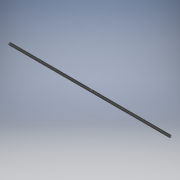
# Autodesk Inventor part: GBN1700MR2-90_info-1-13-13
Saved by Autodesk Inventor 2017.3 (Build 213256000, 256)
## iProperties
Part Number: GBN1700MR2-90_info-1-13-13
Material: Generic
Catalog Web Link: www.cadenas.de
Description: GBN__MR2-High Torque Timing Belts - MR2 Type
Vendor: MISUMI
Document SubType Name: Modeling
Designer: partserver
Manufacturer: MISUMI
Mass: 9.67395 g
Surface Area: 327.945 cm^2
Volume: 9.67395 cm^3
Density: 1 g/cm^3
Appearance: PSOLRGB-175-175-175
Category: PARTsolutions
Company: MISUMI
Title: GBN1700MR2-90
Author: Cadenas PARTsolutions
Comments: High Torque Timing Belts - MR2 Type
PSOL_IDENT_0: {$CADENAS_DATA\23d-libs\misumi\metric\48_timing_belts\gbn_mr2.prj},206 {VTYP=3D},{NB=GBN1700MR2-90_i
PSOL_IDENT_1: nfo-1-13-13},{LINA=GBN1700MR2-90},{NN=GBN__MR2},{DATE=08.06.2021 08:28:53},{GEOMDATE=10.03.2016 05:4
PSOL_IDENT_2: 5:00},{VERSION=},{LINEID=40},{WBVAR=NT,RSSP,NT1,NT2},{WBNUMERIC=NT,NT1,NT2}  {NB=GBN1700MR2-90_info-
PSOL_IDENT_3: 1-13-13},{LINA=GBN1700MR2-90},{KT=DUMMY},{PN=GBN1700MR2-90},{TYPE=GBN},{BNO=1700MR2},{BNW=9},{BNWALG=
PSOL_IDENT_4: 90},{NT=850},{BC=1700},{PITCH=2},{R1=0.15},{R2=1.00},{R3=0.555},{BB=0.40},{H=1.38},{HH=0.75},{II=0.6
PSOL_IDENT_5: 3},{PLD=0.254},{RSSP=1},{RSSPALG= '1','900 or Less','2','Over 900, 1200 or Less','3','Over 1200, 180
PSOL_IDENT_6: 0 or Less','4','Over 1800, 3600 or Less','5','Over 3600, 4800 or Less' },{NT1=13},{NT1ALG=13,14,15,1
PSOL_IDENT_7: 6,17,18,19,20,21,22,24,25,26,28,30,32,34,36,40,42,44,45,48,50,56,60,62,68,72},{NT2=13},{NT2ALG=13,14
PSOL_IDENT_8: ,15,16,17,18,19,20,21,22,24,25,26,28,30,32,34,36,40,42,44,45,48,50,56,60,62,68,72},{NT2ALG1=0},{NT2A
PSOL_IDENT_9: LG2=0},{NT2ALG3=13,14,15,16,17,18,19,20,21,22,24,25,26,28,30,32,34,36,40,42,44,45,48,50,56,60,62,68,
PSOL_IDENT_10: 72},{DRIVEP=8.27606},{DRP=7.77},{DRIVENP=8.27606},{DRNP=7.77},{BBCAL=3348.00000},{C=837.00},{NOTE=-}
PSOL_IDENT_11: ,{ASSCFGC=NT2,C},{ASSCFGCNOTE=-},{FS=0.00},{FL=0.00},{NT1SCR=16,18,20,22,23,24,25,26,28,30,32,34,36,
PSOL_IDENT_12: 40,44,48,50,60},{NT2SCR=0}
NB: GBN1700MR2-90_info-1-13-13
NN: GBN__MR2
NT: 850
NBSYN: $PN._info-$RSSP.-$NT1.-$NT2.
LINA: GBN1700MR2-90
CATALOG: Misumi
PN: GBN1700MR2-90
TYPE: GBN
BNO: 1700MR2
BNW: 9
BC: 1700
PITCH: 2
R1: 0.15
R2: 1
R3: 0.555
BB: 0.4
H: 1.38
HH: 0.75
II: 0.63
PLD: 0.254
RSSP: 900 or Less
NT1: 13
NT2: 13
SUPPLIER: MISUMI
ARTICLENO: GBN1700MR2-90_info-1-13-13
BOMINFO: GBN1700MR2-90
CREATOR: CADENAS GmbH
Autodesk Inventor part; units mm, degrees
ref_plane "YZ Plane" through (0, 0, 0) normal (1, 0, 0) x (0, 1, 0)
ref_plane "XZ Plane" through (0, 0, 0) normal (0, 1, 0) x (-1, 0, 0)
ref_plane "XY Plane" through (0, 0, 0) normal (0, 0, 1) x (1, 0, 0)
sketch "_____1" plane through (0, 0, 0) normal (0, 0, 1) x (1, 0, 0)
  arc A0 (0, 4.515) -> (0, -4.515) centre (0, 0) ccw
  line L0 (0, -4.515) -> (837, -4.515)
  arc A1 (837, -4.515) -> (837, 4.515) centre (837, 0) ccw
  line L1 (837, 4.515) -> (0, 4.515)
  arc A2 (0, 3.885) -> (0, -3.885) centre (0, 0) ccw
  line L2 (0, -3.885) -> (837, -3.885)
  arc A3 (837, -3.885) -> (837, 3.885) centre (837, 0) ccw
  line L3 (837, 3.885) -> (0, 3.885)
  constraints: 8 end point, 8 point on circle, 4 centre point
extrude "Extrusion1" add sketch "_____1" along normal mid plane 9
sketch "_____2" plane through (0, 0, 0) normal (0, 0, 1) x (1, 0, 0)
  line L0 (413.5, 4.515) -> (413.5, 3.885)
  line L1 (413.5, 3.885) -> (413.7598, 3.885)
  arc A0 (413.9085, 3.7546) -> (413.7598, 3.885) centre (413.7598, 3.735) ccw
  arc A1 (413.9085, 3.7546) -> (414.0011, 3.4468) centre (414.9, 3.885) ccw
  arc A2 (414.0011, 3.4468) -> (414.9989, 3.4468) centre (414.5, 3.69) ccw
  arc A3 (414.9989, 3.4468) -> (415.0915, 3.7546) centre (414.1, 3.885) ccw
  arc A4 (415.2402, 3.885) -> (415.0915, 3.7546) centre (415.2402, 3.735) ccw
  line L2 (415.2402, 3.885) -> (415.7598, 3.885)
  arc A5 (415.9085, 3.7546) -> (415.7598, 3.885) centre (415.7598, 3.735) ccw
  arc A6 (415.9085, 3.7546) -> (416.0011, 3.4468) centre (416.9, 3.885) ccw
  arc A7 (416.0011, 3.4468) -> (416.9989, 3.4468) centre (416.5, 3.69) ccw
  arc A8 (416.9989, 3.4468) -> (417.0915, 3.7546) centre (416.1, 3.885) ccw
  arc A9 (417.2402, 3.885) -> (417.0915, 3.7546) centre (417.2402, 3.735) ccw
  line L3 (417.2402, 3.885) -> (417.7598, 3.885)
  arc A10 (417.9085, 3.7546) -> (417.7598, 3.885) centre (417.7598, 3.735) ccw
  arc A11 (417.9085, 3.7546) -> (418.0011, 3.4468) centre (418.9, 3.885) ccw
  arc A12 (418.0011, 3.4468) -> (418.9989, 3.4468) centre (418.5, 3.69) ccw
  arc A13 (418.9989, 3.4468) -> (419.0915, 3.7546) centre (418.1, 3.885) ccw
  arc A14 (419.2402, 3.885) -> (419.0915, 3.7546) centre (419.2402, 3.735) ccw
  line L4 (419.2402, 3.885) -> (419.7598, 3.885)
  arc A15 (419.9085, 3.7546) -> (419.7598, 3.885) centre (419.7598, 3.735) ccw
  arc A16 (419.9085, 3.7546) -> (420.0011, 3.4468) centre (420.9, 3.885) ccw
  arc A17 (420.0011, 3.4468) -> (420.9989, 3.4468) centre (420.5, 3.69) ccw
  arc A18 (420.9989, 3.4468) -> (421.0915, 3.7546) centre (420.1, 3.885) ccw
  arc A19 (421.2402, 3.885) -> (421.0915, 3.7546) centre (421.2402, 3.735) ccw
  line L5 (421.2402, 3.885) -> (421.7598, 3.885)
  arc A20 (421.9085, 3.7546) -> (421.7598, 3.885) centre (421.7598, 3.735) ccw
  arc A21 (421.9085, 3.7546) -> (422.0011, 3.4468) centre (422.9, 3.885) ccw
  arc A22 (422.0011, 3.4468) -> (422.9989, 3.4468) centre (422.5, 3.69) ccw
  arc A23 (422.9989, 3.4468) -> (423.0915, 3.7546) centre (422.1, 3.885) ccw
  arc A24 (423.2402, 3.885) -> (423.0915, 3.7546) centre (423.2402, 3.735) ccw
  line L6 (423.2402, 3.885) -> (423.5, 3.885)
  line L7 (423.5, 3.885) -> (423.5, 4.515)
  line L8 (423.5, 4.515) -> (413.5, 4.515)
  constraints: 50 point on circle, 25 centre point, 18 end point
extrude "Extrusion2" add sketch "_____2" along normal mid plane 9
body "Solid1"
